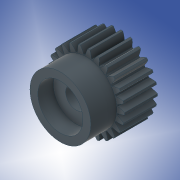
# Autodesk Inventor part: BA012
Saved by Autodesk Inventor 2017 SP1 (Build 210196100, 196)
## iProperties
Created: 2017-06-27
Part Number: BA012
Material: ABS Plastic
Document SubType Name: Modeling
Designer: zallen
Density: 1.06 g/cm^3
Appearance: CR Dark Blue
Author: zallen
Autodesk Inventor part; units mm, degrees
ref_plane "YZ Plane" through (0, 0, 0) normal (1, 0, 0) x (0, 1, 0)
ref_plane "XZ Plane" through (0, 0, 0) normal (0, 1, 0) x (-1, 0, 0)
ref_plane "XY Plane" through (0, 0, 0) normal (0, 0, 1) x (1, 0, 0)
sketch "Sketch1" plane through (0, 0, 0) normal (0, 0, 1) x (1, 0, 0)
  circle A0 centre (0, 0) radius 6
  circle A1 centre (0, 0) radius 18
  dimension "d0" = 12
  dimension "d1" = 36
  constraints: 2 centre point, 2 coincident
  measures "d0" diameter of A0
  measures "d1" diameter of A1
extrude "Extrusion1" add sketch "Sketch1" along normal blind 19
sketch "Sketch2" plane through (0, 0, 19) normal (0, 0, 1) x (1, 0, 0)
  line L0 (0, 0) -> (50.6019, 0) construction
  circle A0 centre (0, 0) radius 18 projected
  arc A1 (21.9098, 0.6) -> (17.9098, 1.8) centre (15.6415, -13.0275) ccw
  arc A2 (17.9098, -1.8) -> (21.9098, -0.6) centre (15.6415, 13.0275) ccw
  arc A3 (21.9098, -0.6) -> (21.9098, 0.6) centre (1.9188, 0) ccw
  arc A4 (17.9098, -1.8) -> (17.9098, 1.8) centre (0, 0) ccw
  arc A5 (21.0722, 6.0299) -> (16.8995, 6.1974) centre (18.3899, -8.7283) ccw
  arc A6 (17.7947, 2.7105) -> (21.3707, 4.8676) centre (11.9103, 16.5081) ccw
  arc A7 (21.3707, 4.8676) -> (21.0722, 6.0299) centre (1.8585, 0.4772) ccw
  arc A8 (17.7947, 2.7105) -> (16.8995, 6.1974) centre (0, 0) ccw
  arc A9 (18.9106, 11.0809) -> (14.8273, 10.2055) centre (19.9828, -3.8807) ccw
  arc A10 (16.5616, 7.0507) -> (19.4887, 10.0293) centre (7.4307, 18.9515) ccw
  arc A11 (19.4887, 10.0293) -> (18.9106, 11.0809) centre (1.6814, 0.9244) ccw
  arc A12 (16.5616, 7.0507) -> (14.8273, 10.2055) centre (0, 0) ccw
  arc A13 (15.5608, 15.4357) -> (11.8235, 13.5722) centre (20.3201, 1.2107) ccw
  arc A14 (14.2878, 10.9479) -> (16.3823, 14.5609) centre (2.4842, 20.204) ccw
  arc A15 (16.3823, 14.5609) -> (15.5608, 15.4357) centre (1.3987, 1.3135) ccw
  arc A16 (14.2878, 10.9479) -> (11.8235, 13.5722) centre (0, 0) ccw
  arc A17 (11.2332, 18.8205) -> (8.0767, 16.0862) centre (19.3806, 6.2261) ccw
  arc A18 (11.1163, 14.1572) -> (12.2464, 18.1775) centre (-2.6183, 20.1871) ccw
  arc A19 (12.2464, 18.1775) -> (11.2332, 18.8205) centre (1.0281, 1.6201) ccw
  arc A20 (11.1163, 14.1572) -> (8.0767, 16.0862) centre (0, 0) ccw
  arc A21 (6.1999, 21.0228) -> (3.8225, 17.5894) centre (17.2234, 10.8502) ccw
  arc A22 (7.2463, 16.477) -> (7.3411, 20.652) centre (-7.5564, 18.9017) ccw
  arc A23 (7.3411, 20.652) -> (6.1999, 21.0228) centre (0.5929, 1.8249) ccw
  arc A24 (7.2463, 16.477) -> (3.8225, 17.5894) centre (0, 0) ccw
  arc A25 (0.7769, 21.9042) -> (-0.6719, 17.9875) centre (13.9839, 14.7927) ccw
  arc A26 (2.921, 17.7614) -> (1.9745, 21.8289) centre (-12.0197, 16.4287) ccw
  arc A27 (1.9745, 21.8289) -> (0.7769, 21.9042) centre (0.1205, 1.915) ccw
  arc A28 (2.921, 17.7614) -> (-0.6719, 17.9875) centre (0, 0) ccw
  arc A29 (-4.6949, 21.4093) -> (-5.1241, 17.2553) centre (9.8658, 17.8056) ccw
  arc A30 (-1.5878, 17.9298) -> (-3.5161, 21.6341) centre (-15.7277, 12.9234) ccw
  arc A31 (-3.5161, 21.6341) -> (-4.6949, 21.4093) centre (-0.3595, 1.8848) ccw
  arc A32 (-1.5878, 17.9298) -> (-5.1241, 17.2553) centre (0, 0) ccw
  arc A33 (-9.8716, 19.5691) -> (-9.2543, 15.4388) centre (5.1278, 19.6997) ccw
  arc A34 (-5.9969, 16.9717) -> (-8.7858, 20.08) centre (-18.4475, 8.606) ccw
  arc A35 (-8.7858, 20.08) -> (-9.8716, 19.5691) centre (-0.817, 1.7362) ccw
  arc A36 (-5.9969, 16.9717) -> (-9.2543, 15.4388) centre (0, 0) ccw
  arc A37 (-14.4281, 16.4993) -> (-12.803, 12.6524) centre (0.0676, 20.356) ccw
  arc A38 (-10.0292, 14.9471) -> (-13.5035, 17.2642) centre (-20.0081, 3.748) ccw
  arc A39 (-13.5035, 17.2642) -> (-14.4281, 16.4993) centre (-1.2231, 1.4784) ccw
  arc A40 (-10.0292, 14.9471) -> (-12.803, 12.6524) centre (0, 0) ccw
  arc A41 (-18.0781, 12.3928) -> (-15.5473, 9.0709) centre (-4.9969, 19.7333) ccw
  arc A42 (-13.4313, 11.9833) -> (-17.3727, 13.3637) centre (-20.3116, -1.3456) ccw
  arc A43 (-17.3727, 13.3637) -> (-18.0781, 12.3928) centre (-1.5523, 1.1278) ccw
  arc A44 (-13.4313, 11.9833) -> (-15.5473, 9.0709) centre (0, 0) ccw
  arc A45 (-20.5921, 7.5077) -> (-17.3147, 4.9194) centre (-9.7474, 17.8707) ccw
  arc A46 (-15.9895, 8.2666) -> (-20.1503, 8.6234) centre (-19.3389, -6.3546) ccw
  arc A47 (-20.1503, 8.6234) -> (-20.5921, 7.5077) centre (-1.784, 0.7063) ccw
  arc A48 (-15.9895, 8.2666) -> (-17.3147, 4.9194) centre (0, 0) ccw
  arc A49 (-21.8122, 2.1508) -> (-17.9941, 0.4589) centre (-13.8854, 14.8852) ccw
  arc A50 (-17.543, 4.0305) -> (-21.6618, 3.3413) centre (-17.151, -10.9644) ccw
  arc A51 (-21.6618, 3.3413) -> (-21.8122, 2.1508) centre (-1.9036, 0.2405) ccw
  arc A52 (-17.543, 4.0305) -> (-17.9941, 0.4589) centre (0, 0) ccw
  arc A53 (-21.6618, -3.3413) -> (-17.543, -4.0305) centre (-17.151, 10.9644) ccw
  arc A54 (-17.9941, -0.4589) -> (-21.8122, -2.1508) centre (-13.8854, -14.8852) ccw
  arc A55 (-21.8122, -2.1508) -> (-21.6618, -3.3413) centre (-1.9036, -0.2405) ccw
  arc A56 (-17.9941, -0.4589) -> (-17.543, -4.0305) centre (0, 0) ccw
  arc A57 (-20.1503, -8.6234) -> (-15.9895, -8.2666) centre (-19.3389, 6.3546) ccw
  arc A58 (-17.3147, -4.9194) -> (-20.5921, -7.5077) centre (-9.7474, -17.8707) ccw
  arc A59 (-20.5921, -7.5077) -> (-20.1503, -8.6234) centre (-1.784, -0.7063) ccw
  arc A60 (-17.3147, -4.9194) -> (-15.9895, -8.2666) centre (0, 0) ccw
  arc A61 (-17.3727, -13.3637) -> (-13.4313, -11.9833) centre (-20.3116, 1.3456) ccw
  arc A62 (-15.5473, -9.0709) -> (-18.0781, -12.3928) centre (-4.9969, -19.7333) ccw
  arc A63 (-18.0781, -12.3928) -> (-17.3727, -13.3637) centre (-1.5523, -1.1278) ccw
  arc A64 (-15.5473, -9.0709) -> (-13.4313, -11.9833) centre (0, 0) ccw
  arc A65 (-13.5035, -17.2642) -> (-10.0292, -14.9471) centre (-20.0081, -3.748) ccw
  arc A66 (-12.803, -12.6524) -> (-14.4281, -16.4993) centre (0.0676, -20.356) ccw
  arc A67 (-14.4281, -16.4993) -> (-13.5035, -17.2642) centre (-1.2231, -1.4784) ccw
  arc A68 (-12.803, -12.6524) -> (-10.0292, -14.9471) centre (0, 0) ccw
  arc A69 (-8.7858, -20.08) -> (-5.9969, -16.9717) centre (-18.4475, -8.606) ccw
  arc A70 (-9.2543, -15.4388) -> (-9.8716, -19.5691) centre (5.1278, -19.6997) ccw
  arc A71 (-9.8716, -19.5691) -> (-8.7858, -20.08) centre (-0.817, -1.7362) ccw
  arc A72 (-9.2543, -15.4388) -> (-5.9969, -16.9717) centre (0, 0) ccw
  arc A73 (-3.5161, -21.6341) -> (-1.5878, -17.9298) centre (-15.7277, -12.9234) ccw
  arc A74 (-5.1241, -17.2553) -> (-4.6949, -21.4093) centre (9.8658, -17.8056) ccw
  arc A75 (-4.6949, -21.4093) -> (-3.5161, -21.6341) centre (-0.3595, -1.8848) ccw
  arc A76 (-5.1241, -17.2553) -> (-1.5878, -17.9298) centre (0, 0) ccw
  arc A77 (1.9745, -21.8289) -> (2.921, -17.7614) centre (-12.0197, -16.4287) ccw
  arc A78 (-0.6719, -17.9875) -> (0.7769, -21.9042) centre (13.9839, -14.7927) ccw
  arc A79 (0.7769, -21.9042) -> (1.9745, -21.8289) centre (0.1205, -1.915) ccw
  arc A80 (-0.6719, -17.9875) -> (2.921, -17.7614) centre (0, 0) ccw
  arc A81 (7.3411, -20.652) -> (7.2463, -16.477) centre (-7.5564, -18.9017) ccw
  arc A82 (3.8225, -17.5894) -> (6.1999, -21.0228) centre (17.2234, -10.8502) ccw
  arc A83 (6.1999, -21.0228) -> (7.3411, -20.652) centre (0.5929, -1.8249) ccw
  arc A84 (3.8225, -17.5894) -> (7.2463, -16.477) centre (0, 0) ccw
  arc A85 (12.2464, -18.1775) -> (11.1163, -14.1572) centre (-2.6183, -20.1871) ccw
  arc A86 (8.0767, -16.0862) -> (11.2332, -18.8205) centre (19.3806, -6.2261) ccw
  arc A87 (11.2332, -18.8205) -> (12.2464, -18.1775) centre (1.0281, -1.6201) ccw
  arc A88 (8.0767, -16.0862) -> (11.1163, -14.1572) centre (0, 0) ccw
  arc A89 (16.3823, -14.5609) -> (14.2878, -10.9479) centre (2.4842, -20.204) ccw
  arc A90 (11.8235, -13.5722) -> (15.5608, -15.4357) centre (20.3201, -1.2107) ccw
  arc A91 (15.5608, -15.4357) -> (16.3823, -14.5609) centre (1.3987, -1.3135) ccw
  arc A92 (11.8235, -13.5722) -> (14.2878, -10.9479) centre (0, 0) ccw
  arc A93 (19.4887, -10.0293) -> (16.5616, -7.0507) centre (7.4307, -18.9515) ccw
  arc A94 (14.8273, -10.2055) -> (18.9106, -11.0809) centre (19.9828, 3.8807) ccw
  arc A95 (18.9106, -11.0809) -> (19.4887, -10.0293) centre (1.6814, -0.9244) ccw
  arc A96 (14.8273, -10.2055) -> (16.5616, -7.0507) centre (0, 0) ccw
  arc A97 (21.3707, -4.8676) -> (17.7947, -2.7105) centre (11.9103, -16.5081) ccw
  arc A98 (16.8995, -6.1974) -> (21.0722, -6.0299) centre (18.3899, 8.7283) ccw
  arc A99 (21.0722, -6.0299) -> (21.3707, -4.8676) centre (1.8585, -0.4772) ccw
  arc A100 (16.8995, -6.1974) -> (17.7947, -2.7105) centre (0, 0) ccw
  point P0 (21.9188, 0)
  point P1 (21.2302, 5.451)
  point P2 (19.2076, 10.5595)
  point P3 (15.9781, 15.0044)
  point P4 (11.7447, 18.5066)
  point P5 (6.7733, 20.846)
  point P6 (1.3763, 21.8755)
  point P7 (-4.1072, 21.5305)
  point P8 (-9.3326, 19.8327)
  point P9 (-13.9716, 16.8887)
  point P10 (-17.7327, 12.8835)
  point P11 (-20.3796, 8.0688)
  point P12 (-21.7459, 2.7472)
  point P13 (-21.7459, -2.7472)
  point P14 (-20.3796, -8.0688)
  point P15 (-17.7327, -12.8835)
  point P16 (-13.9716, -16.8887)
  point P17 (-9.3326, -19.8327)
  point P18 (-4.1072, -21.5305)
  point P19 (1.3763, -21.8755)
  point P20 (6.7733, -20.846)
  point P21 (11.7447, -18.5066)
  point P22 (15.9781, -15.0044)
  point P23 (19.2076, -10.5595)
  point P24 (21.2302, -5.451)
  dimension "d4" = 15
  dimension "d5" = 15
  dimension "d6" = 20
  dimension "d7" = 4
  dimension "d8" = 1.2
  dimension "d9" = 1.8
  dimension "d12" = 360
  constraints: 203 point on circle, 100 centre point, 2 end point, 2 vertical alignment, 1 concentric, 1 horizontal, 1 point on line, 326 other
  measures "d4" radius of A1
  measures "d5" radius of A2
  measures "d6" radius of A3
  measures "d7" horizontal distance of A1.start A0.start
  measures "d8" distance of A2.end A1.start
  measures "d9" distance from line of L0 A0.start
extrude "Extrusion2" add sketch "Sketch2" against normal blind 19 contours A0 A1 A3 A2 | A0 A5 A7 A6 | A97 A99 A98 A0 | A0 A9 A11 A10 | A93 A95 A94 A0 | A0 A13 A15 A14 | A89 A91 A90 A0 | A0 A17 A19 A18 | A85 A87 A86 A0 | A0 A21 A23 A22 | A81 A83 A82 A0 | A0 A25 A27 A26 | A77 A79 A78 A0 | A0 A29 A31 A30 | A73 A75 A74 A0 | A0 A33 A35 A34 | A69 A71 A70 A0 | A0 A37 A39 A38 | A65 A67 A66 A0 | A0 A41 A43 A42 | A61 A63 A62 A0 | A0 A45 A47 A46 | A57 A59 A58 A0 | A0 A49 A51 A50 | A53 A55 A54 A0
sketch "Sketch4" plane through (0, 0, 19) normal (0, 0, 1) x (1, 0, 0)
  circle A0 centre (0, 0) radius 6 projected
  circle A1 centre (0, 0) radius 17.5
  dimension "d19" = 35
  constraints: 1 centre point, 1 coincident
  measures "d19" diameter of A1
extrude "Extrusion4" add sketch "Sketch4" along normal blind 15
sketch "Sketch5" plane through (0, 0, 0) normal (0, 0, -1) x (-1, 0, 0)
  circle A0 centre (0, 0) radius 13
  dimension "d22" = 26
  constraints: 1 centre point, 1 coincident
  measures "d22" diameter of A0
extrude "Extrusion5" cut sketch "Sketch5" against normal blind 9
sketch "Sketch6" plane through (0, 0, 34) normal (0, 0, 1) x (1, 0, 0)
  circle A0 centre (0, 0) radius 13
  dimension "d25" = 26
  constraints: 1 centre point, 1 coincident
  measures "d25" diameter of A0
extrude "Extrusion6" cut sketch "Sketch6" against normal blind 9
body "Solid1"
